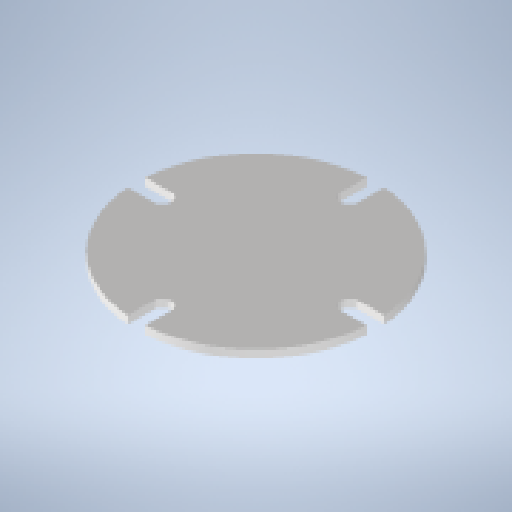
# Autodesk Inventor part: base
Saved by Autodesk Inventor 2025.2 (Build 292293000, 293)
## iProperties
Created: 2025-03-25
Part Number: base
Material: Steel, Mild
Document SubType Name: Modeling
Designer: bless
Density: 7.85 g/cm^3
Appearance: Semi-Polished
Author: bless
Autodesk Inventor part; units mm, degrees
ref_plane "YZ Plane" through (0, 0, 0) normal (1, 0, 0) x (0, 1, 0)
ref_plane "XZ Plane" through (0, 0, 0) normal (0, 1, 0) x (-1, 0, 0)
ref_plane "XY Plane" through (0, 0, 0) normal (0, 0, 1) x (1, 0, 0)
sketch "Sketch1" plane through (0, 0, 0) normal (0, 1, 0) x (-1, 0, 0)
  circle A0 centre (0, 0) radius 150
  circle A1 centre (117.5769, 0) radius 11
  line L0 (117.5769, 11) -> (149.5961, 11)
  line L1 (117.5769, -11) -> (149.5961, -11)
  dimension "d0" = 300
  dimension "d1" = 22
  constraints: 4 end point, 4 point on circle, 2 centre point, 2 tangent, 1 coincident, 1 horizontal, 1 horizontal alignment, 1 parallel
  measures "d0" diameter of A0
  measures "d1" diameter of A1
extrude "Extrusion1" add sketch "Sketch1" along normal blind 10
extrude "Extrusion2" cut sketch "Sketch1" along normal through all contours A0 L1 A1 L0 | A1 picked at (142.3014, 7.7032)
pattern_circular "Circular Pattern1" count 4 over 360 about axis through (0, 0, 0) along (0, 1, 0) of "Extrusion2"
body "Solid1"
